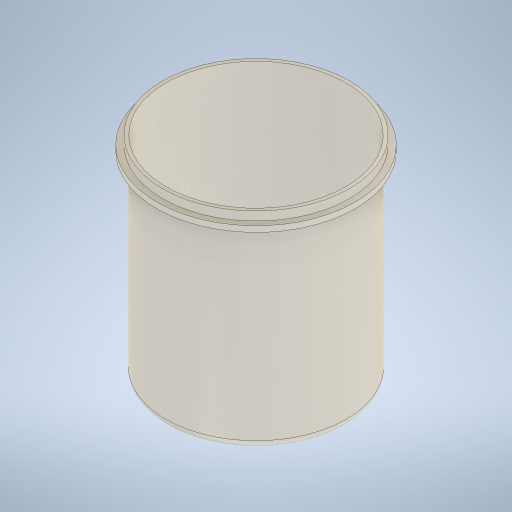
# Autodesk Inventor part: ContenedorTest
Saved by Autodesk Inventor 2024 (Build 280153000, 153)
## iProperties
Created: 2024-05-15
Part Number: ContenedorTest
Material: Genérico
Document SubType Name: Modeling
Designer: alexa
Density: 1 g/cm^3
Appearance: Valor por defecto
Author: alexa
Autodesk Inventor part; units mm, degrees
ref_plane "YZ Plane" through (0, 0, 0) normal (1, 0, 0) x (0, 1, 0)
ref_plane "XZ Plane" through (0, 0, 0) normal (0, 1, 0) x (-1, 0, 0)
ref_plane "XY Plane" through (0, 0, 0) normal (0, 0, 1) x (1, 0, 0)
sketch "Sketch1" plane through (0, 0, 0) normal (0, 0, 1) x (1, 0, 0)
  line L0 (46.8, 0) -> (47, 0)
  line L1 (47, 4.6) -> (47, 101.7)
  line L2 (47, 109.2) -> (46.8, 109.2)
  line L3 (46.8, 109.2) -> (46.8, 4.8)
  line L4 (46.8, 109.2) -> (48.6, 109.2)
  line L5 (48.6, 109.2) -> (48.6, 104.7)
  line L6 (48.6, 104.7) -> (51.6, 104.7)
  line L7 (51.6, 104.7) -> (51.6, 101.7)
  line L8 (51.6, 101.7) -> (48.6, 101.7)
  line L9 (48.6, 101.7) -> (47, 101.7)
  line L10 (0, 0) -> (0, 20.8136)
  line L11 (42.4, 0) -> (-0.2292, 0)
  line L12 (0, 0) -> (0, 0.2)
  line L13 (0, 0.2) -> (42.2, 0.2)
  arc A0 (42.2, 0.2) -> (46.8, 4.8) centre (42.2, 4.8) ccw
  arc A1 (42.4, 0) -> (47, 4.6) centre (42.4, 4.6) ccw
  dimension "d1" = 0.2
  dimension "d2" = 109.2
  dimension "d3" = 1.8
  dimension "d4" = 4.5
  dimension "d5" = 3
  dimension "d6" = 3
  dimension "d7" = 0.2
  dimension "d8" = 90
  dimension "d9" = 4.6
  constraints: 28 end point, 5 perpendicular, 5 point on line, 4 point on circle, 4 tangent, 3 horizontal, 2 centre point, 2 parallel, 1 equal radius, 1 vertical
  measures "d1" distance of L2.end L2.start
  measures "d2" distance of L2.start L0.end
  measures "d3" distance of L2.end L4.end
  measures "d4" distance of L4.end L5.end
  measures "d5" distance of L5.end L6.end
  measures "d6" distance of L6.end L7.end
  measures "d7" distance of L10.start L12.end
  measures "d8" angle of L12 L13
  measures "d9" radius of A0
revolve "Revolution1" add sketch "Sketch1" angle 360 about axis through (0, 0, 0) along (0, 1, 0)
body "Solid1"
